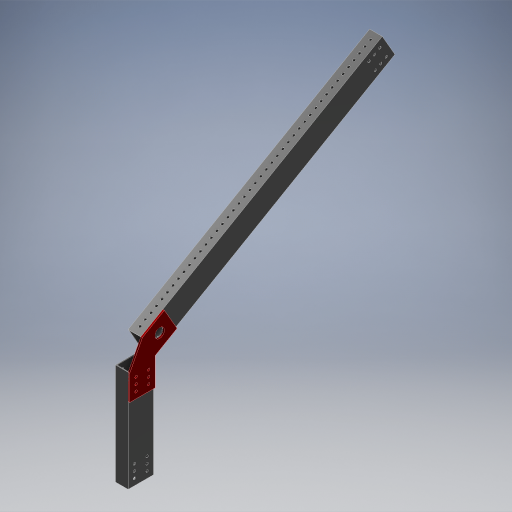
# Autodesk Inventor part: 2024-210-000-Angle-Shootaur
Saved by Autodesk Inventor 2024.2 (Build 282272000, 272)
## iProperties
Created: 2024-01-23
Part Number: 2024-210-000-Angle-Shootaur
Material: Aluminum 6061
Document SubType Name: Modeling
Designer: rohan
Density: 2.7 g/cm^3
Appearance: Aluminum - Flat
Author: rohan
Autodesk Inventor part; units mm, degrees
ref_plane "YZ Plane" through (0, 0, 0) normal (1, 0, 0) x (0, 1, 0)
ref_plane "XZ Plane" through (0, 0, 0) normal (0, 1, 0) x (-1, 0, 0)
ref_plane "XY Plane" through (0, 0, 0) normal (0, 0, 1) x (1, 0, 0)
sketch "Sketch1" plane through (0, 0, 0) normal (1, 0, 0) x (0, 1, 0)
  line L0 (-12.7, 355.6) -> (12.7, 355.6)
  line L1 (12.7, 355.6) -> (12.7, -355.6)
  line L2 (12.7, -355.6) -> (-12.7, -355.6)
  line L3 (-12.7, -355.6) -> (-12.7, 355.6)
  line L4 (-12.7, 355.6) -> (12.7, -355.6) construction
  line L5 (12.7, 355.6) -> (-12.7, -355.6) construction
  line L6 (0, 0) -> (-50.831, 0)
  line L7 (-25.4155, 0) -> (-50.831, 0)
  line L8 (-63.5465, -330.2) -> (-12.7, -330.2)
  line L9 (-12.7, -330.2) -> (-12.7, 330.2)
  line L10 (-12.7, 330.2) -> (-63.5465, 330.2)
  line L11 (-63.5465, 330.2) -> (-63.5465, -330.2)
  line L12 (-63.5465, -330.2) -> (-12.7, 330.2) construction
  line L13 (-12.7, -330.2) -> (-63.5465, 330.2) construction
  circle A0 centre (-25.4, 317.5) radius 2.4892
  circle A1 centre (-38.1, 317.5) radius 2.4892
  circle A2 centre (-50.8, 317.5) radius 2.4892
  circle A3 centre (-25.4, 304.8) radius 2.4892
  circle A4 centre (-38.1, 304.8) radius 2.4892
  circle A5 centre (-50.8, 304.8) radius 2.4892
  circle A6 centre (-25.4, 292.1) radius 2.4892
  circle A7 centre (-38.1, 292.1) radius 2.4892
  circle A8 centre (-50.8, 292.1) radius 2.4892
  circle A9 centre (-25.4, 279.4) radius 2.4892
  circle A10 centre (-38.1, 279.4) radius 2.4892
  circle A11 centre (-50.8, 279.4) radius 2.4892
  circle A12 centre (-25.4, 266.7) radius 2.4892
  circle A13 centre (-38.1, 266.7) radius 2.4892
  circle A14 centre (-50.8, 266.7) radius 2.4892
  circle A15 centre (-25.4, 254) radius 2.4892
  circle A16 centre (-38.1, 254) radius 2.4892
  circle A17 centre (-50.8, 254) radius 2.4892
  circle A18 centre (-25.4, 241.3) radius 2.4892
  circle A19 centre (-38.1, 241.3) radius 2.4892
  circle A20 centre (-50.8, 241.3) radius 2.4892
  circle A21 centre (-25.4, 228.6) radius 2.4892
  circle A22 centre (-38.1, 228.6) radius 2.4892
  circle A23 centre (-50.8, 228.6) radius 2.4892
  circle A24 centre (-25.4, 215.9) radius 2.4892
  circle A25 centre (-38.1, 215.9) radius 2.4892
  circle A26 centre (-50.8, 215.9) radius 2.4892
  circle A27 centre (-25.4, 203.2) radius 2.4892
  circle A28 centre (-38.1, 203.2) radius 2.4892
  circle A29 centre (-50.8, 203.2) radius 2.4892
  circle A30 centre (-25.4, 190.5) radius 2.4892
  circle A31 centre (-38.1, 190.5) radius 2.4892
  circle A32 centre (-50.8, 190.5) radius 2.4892
  circle A33 centre (-25.4, 177.8) radius 2.4892
  circle A34 centre (-38.1, 177.8) radius 2.4892
  circle A35 centre (-50.8, 177.8) radius 2.4892
  circle A36 centre (-25.4, 165.1) radius 2.4892
  circle A37 centre (-38.1, 165.1) radius 2.4892
  circle A38 centre (-50.8, 165.1) radius 2.4892
  circle A39 centre (-25.4, 152.4) radius 2.4892
  circle A40 centre (-38.1, 152.4) radius 2.4892
  circle A41 centre (-50.8, 152.4) radius 2.4892
  circle A42 centre (-25.4, 139.7) radius 2.4892
  circle A43 centre (-38.1, 139.7) radius 2.4892
  circle A44 centre (-50.8, 139.7) radius 2.4892
  circle A45 centre (-25.4, 127) radius 2.4892
  circle A46 centre (-38.1, 127) radius 2.4892
  circle A47 centre (-50.8, 127) radius 2.4892
  circle A48 centre (-25.4, 114.3) radius 2.4892
  circle A49 centre (-38.1, 114.3) radius 2.4892
  circle A50 centre (-50.8, 114.3) radius 2.4892
  circle A51 centre (-25.4, 101.6) radius 2.4892
  circle A52 centre (-38.1, 101.6) radius 2.4892
  circle A53 centre (-50.8, 101.6) radius 2.4892
  circle A54 centre (-25.4, 88.9) radius 2.4892
  circle A55 centre (-38.1, 88.9) radius 2.4892
  circle A56 centre (-50.8, 88.9) radius 2.4892
  circle A57 centre (-25.4, 76.2) radius 2.4892
  circle A58 centre (-38.1, 76.2) radius 2.4892
  circle A59 centre (-50.8, 76.2) radius 2.4892
  circle A60 centre (-25.4, 63.5) radius 2.4892
  circle A61 centre (-38.1, 63.5) radius 2.4892
  circle A62 centre (-50.8, 63.5) radius 2.4892
  circle A63 centre (-25.4, 50.8) radius 2.4892
  circle A64 centre (-38.1, 50.8) radius 2.4892
  circle A65 centre (-50.8, 50.8) radius 2.4892
  circle A66 centre (-25.4, 38.1) radius 2.4892
  circle A67 centre (-38.1, 38.1) radius 2.4892
  circle A68 centre (-50.8, 38.1) radius 2.4892
  circle A69 centre (-25.4, 25.4) radius 2.4892
  circle A70 centre (-38.1, 25.4) radius 2.4892
  circle A71 centre (-50.8, 25.4) radius 2.4892
  circle A72 centre (-25.4, 12.7) radius 2.4892
  circle A73 centre (-38.1, 12.7) radius 2.4892
  circle A74 centre (-50.8, 12.7) radius 2.4892
  circle A75 centre (-25.4, 0) radius 2.4892
  circle A76 centre (-38.1, 0) radius 2.4892
  circle A77 centre (-50.8, 0) radius 2.4892
  circle A78 centre (-25.4, -12.7) radius 2.4892
  circle A79 centre (-38.1, -12.7) radius 2.4892
  circle A80 centre (-50.8, -12.7) radius 2.4892
  circle A81 centre (-25.4, -25.4) radius 2.4892
  circle A82 centre (-38.1, -25.4) radius 2.4892
  circle A83 centre (-50.8, -25.4) radius 2.4892
  circle A84 centre (-25.4, -38.1) radius 2.4892
  circle A85 centre (-38.1, -38.1) radius 2.4892
  circle A86 centre (-50.8, -38.1) radius 2.4892
  circle A87 centre (-25.4, -50.8) radius 2.4892
  circle A88 centre (-38.1, -50.8) radius 2.4892
  circle A89 centre (-50.8, -50.8) radius 2.4892
  circle A90 centre (-25.4, -63.5) radius 2.4892
  circle A91 centre (-38.1, -63.5) radius 2.4892
  circle A92 centre (-50.8, -63.5) radius 2.4892
  circle A93 centre (-25.4, -76.2) radius 2.4892
  circle A94 centre (-38.1, -76.2) radius 2.4892
  circle A95 centre (-50.8, -76.2) radius 2.4892
  circle A96 centre (-25.4, -88.9) radius 2.4892
  circle A97 centre (-38.1, -88.9) radius 2.4892
  circle A98 centre (-50.8, -88.9) radius 2.4892
  circle A99 centre (-25.4, -101.6) radius 2.4892
  circle A100 centre (-38.1, -101.6) radius 2.4892
  circle A101 centre (-50.8, -101.6) radius 2.4892
  circle A102 centre (-25.4, -114.3) radius 2.4892
  circle A103 centre (-38.1, -114.3) radius 2.4892
  circle A104 centre (-50.8, -114.3) radius 2.4892
  circle A105 centre (-25.4, -127) radius 2.4892
  circle A106 centre (-38.1, -127) radius 2.4892
  circle A107 centre (-50.8, -127) radius 2.4892
  circle A108 centre (-25.4, -139.7) radius 2.4892
  circle A109 centre (-38.1, -139.7) radius 2.4892
  circle A110 centre (-50.8, -139.7) radius 2.4892
  circle A111 centre (-25.4, -152.4) radius 2.4892
  circle A112 centre (-38.1, -152.4) radius 2.4892
  circle A113 centre (-50.8, -152.4) radius 2.4892
  circle A114 centre (-25.4, -165.1) radius 2.4892
  circle A115 centre (-38.1, -165.1) radius 2.4892
  circle A116 centre (-50.8, -165.1) radius 2.4892
  circle A117 centre (-25.4, -177.8) radius 2.4892
  circle A118 centre (-38.1, -177.8) radius 2.4892
  circle A119 centre (-50.8, -177.8) radius 2.4892
  circle A120 centre (-25.4, -190.5) radius 2.4892
  circle A121 centre (-38.1, -190.5) radius 2.4892
  circle A122 centre (-50.8, -190.5) radius 2.4892
  circle A123 centre (-25.4, -203.2) radius 2.4892
  circle A124 centre (-38.1, -203.2) radius 2.4892
  circle A125 centre (-50.8, -203.2) radius 2.4892
  circle A126 centre (-25.4, -215.9) radius 2.4892
  circle A127 centre (-38.1, -215.9) radius 2.4892
  circle A128 centre (-50.8, -215.9) radius 2.4892
  circle A129 centre (-25.4, -228.6) radius 2.4892
  circle A130 centre (-38.1, -228.6) radius 2.4892
  circle A131 centre (-50.8, -228.6) radius 2.4892
  circle A132 centre (-25.4, -241.3) radius 2.4892
  circle A133 centre (-38.1, -241.3) radius 2.4892
  circle A134 centre (-50.8, -241.3) radius 2.4892
  circle A135 centre (-25.4, -254) radius 2.4892
  circle A136 centre (-38.1, -254) radius 2.4892
  circle A137 centre (-50.8, -254) radius 2.4892
  circle A138 centre (-25.4, -266.7) radius 2.4892
  circle A139 centre (-38.1, -266.7) radius 2.4892
  circle A140 centre (-50.8, -266.7) radius 2.4892
  circle A141 centre (-25.4, -279.4) radius 2.4892
  circle A142 centre (-38.1, -279.4) radius 2.4892
  circle A143 centre (-50.8, -279.4) radius 2.4892
  circle A144 centre (-25.4, -292.1) radius 2.4892
  circle A145 centre (-38.1, -292.1) radius 2.4892
  circle A146 centre (-50.8, -292.1) radius 2.4892
  circle A147 centre (0, 342.9) radius 2.4892
  circle A148 centre (0, 330.2) radius 2.4892
  circle A149 centre (0, 317.5) radius 2.4892
  circle A150 centre (0, 304.8) radius 2.4892
  circle A151 centre (0, 292.1) radius 2.4892
  circle A152 centre (0, 279.4) radius 2.4892
  circle A153 centre (0, 266.7) radius 2.4892
  circle A154 centre (0, 254) radius 2.4892
  circle A155 centre (0, 241.3) radius 2.4892
  circle A156 centre (0, 228.6) radius 2.4892
  circle A157 centre (0, 215.9) radius 2.4892
  circle A158 centre (0, 203.2) radius 2.4892
  circle A159 centre (0, 190.5) radius 2.4892
  circle A160 centre (0, 177.8) radius 2.4892
  circle A161 centre (0, 165.1) radius 2.4892
  circle A162 centre (0, 152.4) radius 2.4892
  circle A163 centre (0, 139.7) radius 2.4892
  circle A164 centre (0, 127) radius 2.4892
  circle A165 centre (0, 114.3) radius 2.4892
  circle A166 centre (0, 101.6) radius 2.4892
  circle A167 centre (0, 88.9) radius 2.4892
  circle A168 centre (0, 76.2) radius 2.4892
  circle A169 centre (0, 63.5) radius 2.4892
  circle A170 centre (0, 50.8) radius 2.4892
  circle A171 centre (0, 38.1) radius 2.4892
  circle A172 centre (0, 25.4) radius 2.4892
  circle A173 centre (0, 12.7) radius 2.4892
  circle A174 centre (0, 0) radius 2.4892
  circle A175 centre (0, -12.7) radius 2.4892
  circle A176 centre (0, -25.4) radius 2.4892
  circle A177 centre (0, -38.1) radius 2.4892
  circle A178 centre (0, -50.8) radius 2.4892
  circle A179 centre (0, -63.5) radius 2.4892
  circle A180 centre (0, -76.2) radius 2.4892
  circle A181 centre (0, -88.9) radius 2.4892
  circle A182 centre (0, -101.6) radius 2.4892
  circle A183 centre (0, -114.3) radius 2.4892
  circle A184 centre (0, -127) radius 2.4892
  circle A185 centre (0, -139.7) radius 2.4892
  circle A186 centre (0, -152.4) radius 2.4892
  circle A187 centre (0, -165.1) radius 2.4892
  circle A188 centre (0, -177.8) radius 2.4892
  circle A189 centre (0, -190.5) radius 2.4892
  circle A190 centre (0, -203.2) radius 2.4892
  circle A191 centre (0, -215.9) radius 2.4892
  circle A192 centre (0, -228.6) radius 2.4892
  circle A193 centre (0, -241.3) radius 2.4892
  circle A194 centre (0, -254) radius 2.4892
  circle A195 centre (0, -266.7) radius 2.4892
  circle A196 centre (0, -279.4) radius 2.4892
  circle A197 centre (0, -292.1) radius 2.4892
  circle A198 centre (0, -304.8) radius 2.4892
  circle A199 centre (0, -317.5) radius 2.4892
  line L14 (12.7, 254) -> (215.9, 254)
  line L15 (215.9, 254) -> (215.9, 203.2)
  line L16 (215.9, 203.2) -> (12.7, 203.2)
  line L17 (12.7, 203.2) -> (12.7, 254)
  line L18 (12.7, -76.2) -> (292.1, -76.2)
  line L19 (292.1, -76.2) -> (292.1, -127)
  line L20 (292.1, -127) -> (12.7, -127)
  line L21 (12.7, -127) -> (12.7, -76.2)
  line L22 (544.3741, -255.335) -> (500.38, -280.735)
  line L23 (500.38, -280.735) -> (220.98, 203.2)
  line L24 (220.98, 203.2) -> (264.9741, 228.6)
  line L25 (264.9741, 228.6) -> (544.3741, -255.335)
  circle A200 centre (203.2, 241.3) radius 2.4892
  circle A201 centre (203.2, 215.9) radius 2.4892
  circle A202 centre (190.5, 241.3) radius 2.4892
  circle A203 centre (190.5, 215.9) radius 2.4892
  circle A204 centre (177.8, 241.3) radius 2.4892
  circle A205 centre (177.8, 215.9) radius 2.4892
  line L26 (114.3, 254) -> (114.3, 203.2) construction
  circle A206 centre (25.4, 241.3) radius 2.4892
  circle A207 centre (25.4, 215.9) radius 2.4892
  circle A208 centre (38.1, 241.3) radius 2.4892
  circle A209 centre (38.1, 215.9) radius 2.4892
  circle A210 centre (50.8, 241.3) radius 2.4892
  circle A211 centre (50.8, 215.9) radius 2.4892
  circle A212 centre (255.677, 193.903) radius 9.525
  circle A213 centre (279.4, -88.9) radius 2.4892
  circle A214 centre (279.4, -114.3) radius 2.4892
  circle A215 centre (266.7, -88.9) radius 2.4892
  circle A216 centre (266.7, -114.3) radius 2.4892
  circle A217 centre (254, -88.9) radius 2.4892
  circle A218 centre (254, -114.3) radius 2.4892
  line L27 (152.4, -76.2) -> (152.4, -127) construction
  circle A219 centre (25.4, -88.9) radius 2.4892
  circle A220 centre (25.4, -114.3) radius 2.4892
  circle A221 centre (38.1, -88.9) radius 2.4892
  circle A222 centre (38.1, -114.3) radius 2.4892
  circle A223 centre (50.8, -88.9) radius 2.4892
  circle A224 centre (50.8, -114.3) radius 2.4892
  circle A225 centre (527.0256, -250.6865) radius 2.4892
  circle A226 centre (505.0285, -263.3865) radius 2.4892
  circle A227 centre (520.6756, -239.688) radius 2.4892
  circle A228 centre (498.6785, -252.388) radius 2.4892
  circle A229 centre (514.3256, -228.6894) radius 2.4892
  circle A230 centre (492.3285, -241.3894) radius 2.4892
  line L28 (220.98, 203.2) -> (220.98, 152.4)
  line L29 (74.3982, -401.7115) -> (51.378, -390.977)
  line L30 (51.378, -390.977) -> (188.3926, -97.1481)
  line L31 (188.3926, -97.1481) -> (211.4128, -107.8826)
  line L32 (211.4128, -107.8826) -> (74.3982, -401.7115)
  line L33 (188.3926, -97.1481) -> (188.3926, -149.6965)
  point P0 (-38.1233, 0)
  point P1 (0, 355.6)
  point P2 (12.7, 203.2)
  point P3 (12.7, -127)
  dimension "d0" = 25.4
  dimension "d1" = 711.2
  dimension "d3" = 660.4
  dimension "d4" = 4.9784
  dimension "d5" = 12.7
  dimension "d6" = 12.7
  dimension "d9" = 12.7
  dimension "d12" = 12.7
  dimension "d15" = 4.9784
  dimension "d16" = 12.7
  dimension "d17" = 12.7
  dimension "d20" = 12.7
  dimension "d25" = 203.2
  dimension "d26" = 50.8
  dimension "d28" = 50.8
  dimension "d29" = 50.8
  dimension "d31" = 101.6
  dimension "d34" = 5.08
  dimension "d37" = 558.8
  dimension "d38" = 279.4
  dimension "d39" = 4.9784
  dimension "d40" = 12.7
  dimension "d41" = 12.7
  dimension "d44" = 25.4
  dimension "d47" = 12.7
  dimension "d50" = 19.05
  dimension "d51" = 4.9784
  dimension "d52" = 12.7
  dimension "d53" = 12.7
  dimension "d56" = 25.4
  dimension "d59" = 12.7
  dimension "d62" = 4.9784
  dimension "d63" = 12.7
  dimension "d64" = 12.7
  dimension "d67" = 25.4
  dimension "d70" = 12.7
  dimension "d79" = 30
  dimension "d80" = 25.4
  dimension "d81" = 25.4
  dimension "d105" = 228.6
  dimension "d106" = 25.4
  dimension "d107" = -25
  constraints: 231 centre point, 68 end point, 12 parallel, 12 symmetric about line, 11 midpoint, 8 horizontal, 6 perpendicular, 6 vertical, 3 point on line, 1 collinear, 440 other
  measures "d0" distance of L1.end L2.end
  measures "d1" distance of L0.end L1.end
  measures "d3" distance of L9.end L8.end
  measures "d4" diameter of A0
  measures "d5" distance from line of L3 A0.centre
  measures "d6" distance from line of L10 A0.centre
  measures "d9" distance of A0.centre A1.centre
  measures "d12" distance of A0.centre A3.centre
  measures "d15" diameter of A147
  measures "d16" distance of point (0, 355.6) A147.centre
  measures "d17" distance from line of L1 A147.centre
  measures "d20" distance of A147.centre A148.centre
  measures "d25" distance of L15.end L16.end
  measures "d26" distance of L14.end L15.end
  measures "d28" distance of L18.end L19.end
  measures "d29" distance of L22.start L22.end
  measures "d31" distance between parallel lines of L14 L0
  measures "d34" distance of L23.end L15.end
  measures "d37" distance between parallel lines of L24 L22
  measures "d38" distance of L19.end L20.end
  measures "d39" diameter of A200
  measures "d40" distance from line of L15 A200.centre
  measures "d41" distance from line of L14 A200.centre
  measures "d44" distance of A200.centre A201.centre
  measures "d47" distance of A200.centre A202.centre
  measures "d50" diameter of A212
  measures "d51" diameter of A213
  measures "d52" distance from line of L19 A213.centre
  measures "d53" distance from line of L18 A213.centre
  measures "d56" distance of A213.centre A214.centre
  measures "d59" distance of A213.centre A215.centre
  measures "d62" diameter of A225
  measures "d63" distance from line of L22 A225.centre
  measures "d64" distance from line of L25 A225.centre
  measures "d67" distance of A225.centre A226.centre
  measures "d70" distance of A225.centre A227.centre
  measures "d79" angle of L23 L28
  measures "d80" distance from line of L23 A212.centre
  measures "d81" distance from line of L24 A212.centre
  measures "d105" distance between parallel lines of L2 L20
  measures "d106" distance of L29.start L29.end
  measures "d107" angle of L33 L30
extrude "Extrusion1" add sketch "Sketch1" against normal blind 25.4 contours L14 L15 L16 L1
extrude "Extrusion2" add sketch "Sketch1" against normal blind 25.4 separate body contours L22 L23 L24 L25
sketch "Sketch3" plane through (-25.4, 500.38, -280.735) normal (0, 0.5, -0.866) x (1, 0, 0)
  line L0 (25.4, 0) -> (25.4, -50.8) projected
  line L1 (25.4, 0) -> (0, 0) projected
  line L2 (0, -50.8) -> (0, 0) projected
  line L3 (25.4, -50.8) -> (0, -50.8) projected
  line L4 (23.8125, -49.2125) -> (23.8125, -1.5875)
  line L5 (23.8125, -1.5875) -> (1.5875, -1.5875)
  line L6 (1.5875, -1.5875) -> (1.5875, -49.2125)
  line L7 (1.5875, -49.2125) -> (23.8125, -49.2125)
  point P0 (25.4, 292.9743)
  dimension "d86" = 1.5875
  constraints: 8 end point, 3 other
  measures "d86" distance between parallel lines of L0 L4
extrude "Extrusion5" cut sketch "Sketch3" against normal up to surface (558.8 mm away) contours L7 L6 L5 L4 bodies 2
sketch "Sketch4" plane through (0, 215.9, 254) normal (0, 1, 0) x (1, 0, 0)
  line L0 (0, 50.8) -> (0, 0) projected
  line L1 (0, 50.8) -> (-25.4, 50.8) projected
  line L2 (-25.4, 0) -> (-25.4, 50.8) projected
  line L3 (0, 0) -> (-25.4, 0) projected
  line L4 (-23.8125, 49.2125) -> (-1.5875, 49.2125)
  line L5 (-1.5875, 49.2125) -> (-1.5875, 1.5875)
  line L6 (-1.5875, 1.5875) -> (-23.8125, 1.5875)
  line L7 (-23.8125, 1.5875) -> (-23.8125, 49.2125)
  point P0 (0, 254)
  dimension "d89" = 1.5875
  constraints: 8 end point, 3 other
  measures "d89" distance between parallel lines of L2 L7
extrude "Extrusion6" cut sketch "Sketch4" against normal through all contours L4 L5 L6 L7 bodies 1
sketch "Sketch5" plane through (-25.4, 544.3741, -255.335) normal (0, 0.866, 0.5) x (1, 0, 0)
  line L0 (25.4, 0) -> (25.4, -558.8) projected
  line L1 (25.4, 0) -> (0, 0) projected
  line L2 (0, -558.8) -> (0, 0) projected
  line L3 (25.4, -558.8) -> (0, -558.8) projected
  circle A0 centre (12.7, -546.1) radius 2.4892
  circle A1 centre (12.7, -533.4) radius 2.4892
  circle A2 centre (12.7, -520.7) radius 2.4892
  circle A3 centre (12.7, -508) radius 2.4892
  circle A4 centre (12.7, -495.3) radius 2.4892
  circle A5 centre (12.7, -482.6) radius 2.4892
  circle A6 centre (12.7, -469.9) radius 2.4892
  circle A7 centre (12.7, -457.2) radius 2.4892
  circle A8 centre (12.7, -444.5) radius 2.4892
  circle A9 centre (12.7, -431.8) radius 2.4892
  circle A10 centre (12.7, -419.1) radius 2.4892
  circle A11 centre (12.7, -406.4) radius 2.4892
  circle A12 centre (12.7, -393.7) radius 2.4892
  circle A13 centre (12.7, -381) radius 2.4892
  circle A14 centre (12.7, -368.3) radius 2.4892
  circle A15 centre (12.7, -355.6) radius 2.4892
  circle A16 centre (12.7, -342.9) radius 2.4892
  circle A17 centre (12.7, -330.2) radius 2.4892
  circle A18 centre (12.7, -317.5) radius 2.4892
  circle A19 centre (12.7, -304.8) radius 2.4892
  circle A20 centre (12.7, -292.1) radius 2.4892
  circle A21 centre (12.7, -279.4) radius 2.4892
  circle A22 centre (12.7, -266.7) radius 2.4892
  circle A23 centre (12.7, -254) radius 2.4892
  circle A24 centre (12.7, -241.3) radius 2.4892
  circle A25 centre (12.7, -228.6) radius 2.4892
  circle A26 centre (12.7, -215.9) radius 2.4892
  circle A27 centre (12.7, -203.2) radius 2.4892
  circle A28 centre (12.7, -190.5) radius 2.4892
  circle A29 centre (12.7, -177.8) radius 2.4892
  circle A30 centre (12.7, -165.1) radius 2.4892
  circle A31 centre (12.7, -152.4) radius 2.4892
  circle A32 centre (12.7, -139.7) radius 2.4892
  circle A33 centre (12.7, -127) radius 2.4892
  circle A34 centre (12.7, -114.3) radius 2.4892
  circle A35 centre (12.7, -101.6) radius 2.4892
  circle A36 centre (12.7, -88.9) radius 2.4892
  circle A37 centre (12.7, -76.2) radius 2.4892
  circle A38 centre (12.7, -63.5) radius 2.4892
  circle A39 centre (12.7, -50.8) radius 2.4892
  circle A40 centre (12.7, -38.1) radius 2.4892
  circle A41 centre (12.7, -25.4) radius 2.4892
  circle A42 centre (12.7, -12.7) radius 2.4892
  point P0 (25.4, -493.3136)
  dimension "d92" = 4.9784
  dimension "d93" = 12.7
  dimension "d94" = 12.7
  dimension "d97" = 12.7
  constraints: 43 centre point, 1 vertical, 84 other
  measures "d92" diameter of A0
  measures "d93" distance from line of L3 A0.centre
  measures "d94" distance from line of L2 A0.centre
  measures "d97" distance of A0.centre A1.centre
extrude "Extrusion7" cut sketch "Sketch5" against normal blind 50.8 contours A0 | A1 | A2 | A3 | A4 | A5 | A6 | A7 | A8 | A9 | A10 | A11 | A12 | A13 | A14 | A15 | A16 | A17 | A18 | A19 | A20 | A21 | A22 | A23 | A24 | A25 | A26 | A27 | A28 | A29 | A30 | A31 | A32 | A33 | A34 | A35 | A36 | A37 | A38 | A39 | A40 | A41 | A42 bodies 2
sketch "Sketch6" plane through (0, 0, 0) normal (1, 0, 0) x (0, 0, -1)
  line L0 (-254, 215.9) -> (-254, 12.7) projected
  line L1 (-254, 12.7) -> (-203.2, 12.7) projected
  line L2 (-203.2, 12.7) -> (-203.2, 215.9) projected
  line L3 (-203.2, 215.9) -> (-254, 215.9) projected
  circle A0 centre (-241.3, 25.4) radius 2.4892 projected
  circle A1 centre (-241.3, 38.1) radius 2.4892 projected
  circle A2 centre (-241.3, 50.8) radius 2.4892 projected
  circle A3 centre (-215.9, 177.8) radius 2.4892 projected
  circle A4 centre (-215.9, 190.5) radius 2.4892 projected
  circle A5 centre (-215.9, 203.2) radius 2.4892 projected
  circle A6 centre (-241.3, 203.2) radius 2.4892 projected
  circle A7 centre (-241.3, 190.5) radius 2.4892 projected
  circle A8 centre (-241.3, 177.8) radius 2.4892 projected
  circle A9 centre (-215.9, 50.8) radius 2.4892 projected
  circle A10 centre (-215.9, 38.1) radius 2.4892 projected
  circle A11 centre (-215.9, 25.4) radius 2.4892 projected
  line L4 (-228.6, 264.9741) -> (-203.2, 220.98) projected
  line L5 (-203.2, 220.98) -> (280.735, 500.38) projected
  line L6 (280.735, 500.38) -> (255.335, 544.3741) projected
  line L7 (255.335, 544.3741) -> (-228.6, 264.9741) projected
  circle A12 centre (241.3894, 492.3285) radius 2.4892 projected
  circle A13 centre (228.6894, 514.3256) radius 2.4892 projected
  circle A14 centre (252.388, 498.6785) radius 2.4892 projected
  circle A15 centre (239.688, 520.6756) radius 2.4892 projected
  circle A16 centre (263.3865, 505.0285) radius 2.4892 projected
  circle A17 centre (250.6865, 527.0256) radius 2.4892 projected
  circle A18 centre (-193.903, 255.677) radius 9.525 projected
  line L8 (-203.2, 215.9) -> (-203.2, 220.98)
  line L9 (-254, 215.9) -> (-228.6, 264.9741)
  line L10 (-228.6, 264.9741) -> (-184.6059, 290.3741)
  line L11 (-184.6059, 290.3741) -> (-159.2059, 246.38)
  line L12 (-254, 215.9) -> (-254, 165.1)
  line L13 (-254, 165.1) -> (-203.2, 165.1)
  point P0 (0, 0)
  dimension "d108" = 50.8
  dimension "d109" = 50.8
  constraints: 12 end point, 4 point on line, 2 perpendicular
  measures "d108" distance of L4.start L10.end
  measures "d109" distance of L0.start L12.end
extrude "Extrusion8" add sketch "Sketch6" along normal blind 3.175 separate body contours L3 L2 L13 L0 | L9 L4 L8 L3 | L7 L11 L5 L4
